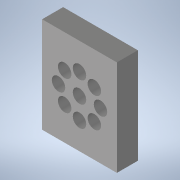
# Autodesk Inventor part: Foam_Top_Big_Mic
Saved by Autodesk Inventor 2021 (Build 250183000, 183)
## iProperties
Created: 2021-02-18
Part Number: Foam_Top_Big_Mic
Material: Polystyrene, Expanded
Document SubType Name: Modeling
Designer: negt20
Density: 0.05 g/cm^3
Appearance: Gray
Author: negt20
Autodesk Inventor part; units mm, degrees
ref_plane "YZ Plane" through (0, 0, 0) normal (1, 0, 0) x (0, 1, 0)
ref_plane "XZ Plane" through (0, 0, 0) normal (0, 1, 0) x (-1, 0, 0)
ref_plane "XY Plane" through (0, 0, 0) normal (0, 0, 1) x (1, 0, 0)
sketch "Sketch1" plane through (0, 0, 0) normal (0, 0, 1) x (1, 0, 0)
  line L0 (-50, 57) -> (50, 57)
  line L1 (50, 57) -> (50, -57)
  line L2 (50, -57) -> (-50, -57)
  line L3 (-50, -57) -> (-50, 57)
  point P0 (0, 0)
  point P1 (0, 57)
  point P2 (-50, 0)
  dimension "d0" = 100
  dimension "d1" = 114
  constraints: 8 end point, 2 midpoint, 2 parallel, 1 horizontal, 1 horizontal alignment, 1 perpendicular, 1 vertical alignment
  measures "d0" distance of L1.end L2.end
  measures "d1" distance of L0.end L1.end
extrude "Extrusion1" add sketch "Sketch1" along normal blind 25
sketch "Sketch2" plane through (0, 0, 0) normal (0, 0, -1) x (-1, 0, 0)
  line L0 (50, -57) -> (-50, -57) projected
  line L1 (-50, 57) -> (50, 57) projected
  line L2 (-50, -57) -> (50, 57) construction
  circle A0 centre (0, 0) radius 8
  line L3 (0, 0) -> (-25, 0) construction
  circle A1 centre (-25, 0) radius 8
  dimension "d4" = 16
  dimension "d5" = 25
  dimension "d6" = 16
  constraints: 4 end point, 2 centre point, 2 coincident, 1 horizontal
  measures "d4" diameter of A0
  measures "d5" distance of L3.start L3.end
  measures "d6" diameter of A1
extrude "Extrusion2" cut sketch "Sketch2" against normal through all
pattern_circular "Circular Pattern1" count 8 over 360 about axis through (0, 0, 0) along (0, 0, 1) of "Extrusion2"
body "Solid1"
